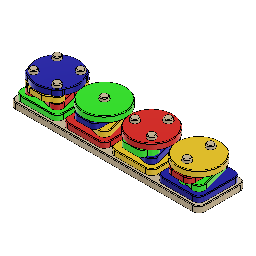
SHAPESpuzzle (Autodesk Fusion 360 design; units mm, degrees)
Autodesk Fusion 360 part; units mm, degrees
note: some values were not read from the file. Chosen so that the rebuilt part matches the saved one: which pieces of a blend or face edit are solid. Set by a fixed rule: which sketch regions a step uses.
sketch "baseboard" plane through (0, 0, 0) normal (0, 0, 1) x (1, 0, 0) in component "base"
  line L0 (160, 40) -> (-160, 40)
  line L1 (-160, 40) -> (-160, -40)
  line L2 (-160, -40) -> (160, -40)
  line L3 (160, -40) -> (160, 40)
  line L4 (160, 40) -> (-160, -40) construction
  line L5 (-160, 40) -> (160, -40) construction
  line L6 (80, 40) -> (-80, 40) construction
  line L7 (-80, 40) -> (-80, -40) construction
  line L8 (-80, -40) -> (80, -40) construction
  line L9 (80, -40) -> (80, 40) construction
  line L10 (80, 40) -> (-80, -40) construction
  line L11 (-80, 40) -> (80, -40) construction
  line L12 (0, 40) -> (0, -40) construction
  line L13 (80, 40) -> (160, -40) construction
  line L14 (160, 40) -> (80, -40) construction
  line L15 (80, -40) -> (0, 40) construction
  line L16 (0, 40) -> (-80, -40) construction
  line L17 (-80, -40) -> (-160, 40) construction
  line L18 (-160, -40) -> (-80, 40) construction
  line L19 (-80, 40) -> (0, -40) construction
  line L20 (0, -40) -> (80, 40) construction
  circle A0 centre (-40, 0) radius 6
  line L21 (120, 40) -> (120, -40)
  circle A1 centre (120, 20) radius 6
  circle A2 centre (120, -20) radius 6
  circle A3 centre (-100, -20) radius 6
  circle A4 centre (-100, 20) radius 6
  circle A5 centre (-140, 20) radius 6
  circle A6 centre (-140, -20) radius 6
  circle A7 centre (56.3299, -16.3299) radius 6
  circle A8 centre (45.9772, 22.3071) radius 6
  circle A9 centre (17.6929, -5.9772) radius 6
  point P0 (120, 0)
  point P1 (-120, 0)
  point P2 (40, 0)
  dimension "d1" = 320
  dimension "d2" = 80
  dimension "d3" = 160
  dimension "d4" = 80
  dimension "d7" = 12
  dimension "d8" = 40
  dimension "d9" = 12
  dimension "d11" = 20
  dimension "d13" = 360
  dimension "d26" = 12
  dimension "d27" = 28.2843
  dimension "d29" = 360
  dimension "d89" = 12
  dimension "d90" = 23.094
  dimension "d92" = 360
  constraint horizontal L0
  constraint perpendicular L0 L1
  constraint parallel L0 L2
  constraint parallel L1 L3
  constraint coincident L4 origin
  constraint coincident L5 origin
  constraint horizontal L6
  constraint perpendicular L6 L7
  constraint parallel L6 L8
  constraint parallel L7 L9
  constraint coincident L10 origin
  constraint coincident L11 origin
  constraint midpoint L0 L12.start
  constraint midpoint L2 L12.end
  constraint midpoint L19 A0.centre
  constraint coincident L0 L21.start
  constraint coincident L2 L21.end
  constraint perpendicular L2 L21
  constraint coincident L21 A1.centre
  constraint midpoint L13 P0
  constraint midpoint L17 P1
  constraint midpoint L15 P2
  constraint coincident L17 A3.centre
  constraint coincident L15 A7.centre
  measures "d1" distance of L1.end L2.end
  measures "d2" distance of L0.end L1.end
  measures "d3" distance of L7.end L8.end
  measures "d4" distance of L6.end L7.end
  measures "d7" diameter of A0
  measures "d8" distance of L6.start L21.start
  measures "d9" diameter of A1
  measures "d11" distance of A1.centre P0
  measures "d26" diameter of A3
  measures "d27" distance of P1 A3.centre
  measures "d89" diameter of A7
  measures "d90" distance of P2 A7.centre
extrude "Extrude1" add sketch "baseboard" along normal blind 10 contours L0 L2 L3 L21 A1 A2 | L0 L1 L2 L21 A1 A2 makes body 1 in component "base"
fillet "Fillet1" radius 10 4 edges at (-160, 40, 5) (-160, -40, 5) (160, -40, 5) (160, 40, 5) on bodies 1 in component "base"
ref_plane "WorkPlane2" through (0, 0, -40) normal (0, 0, 1) x (1, 0, 0) in component "base"
sketch "laser cutting" plane through (0, 0, -40) normal (0, 0, 1) x (1, 0, 0) in component "base"
  arc A0 (160, 30) -> (150, 40) centre (150, 30) ccw
  line L0 (150, 40) -> (-150, 40)
  arc A1 (-150, 40) -> (-160, 30) centre (-150, 30) ccw
  line L1 (-160, 30) -> (-160, -30)
  arc A2 (-160, -30) -> (-150, -40) centre (-150, -30) ccw
  line L2 (-150, -40) -> (150, -40)
  arc A3 (150, -40) -> (160, -30) centre (150, -30) ccw
  line L3 (160, -30) -> (160, 30)
  circle A4 centre (-100, 20) radius 6
  circle A5 centre (-40, 0) radius 6
  circle A6 centre (-140, 20) radius 6
  circle A7 centre (120, -20) radius 6
  circle A8 centre (120, 20) radius 6
  circle A9 centre (-100, -20) radius 6
  circle A10 centre (-140, -20) radius 6
  circle A11 centre (17.6929, -5.9772) radius 6
  circle A12 centre (45.9772, 22.3071) radius 6
  circle A13 centre (56.3299, -16.3299) radius 6
chamfer "Chamfer2" distance 1 angle 45 8 edges at (160, 0, 10) (157.0711, 37.0711, 10) (0, 40, 10) (-157.0711, 37.0711, 10) (-160, 0, 10) (-157.0711, -37.0711, 10) (0, -40, 10) (157.0711, -37.0711, 10) on bodies 1 in component "base"
extrude "Extrude1'" add sketch "baseboard" along normal blind 55 separate body contours L21 A1 | L21 A1 | L21 A2 | L21 A2 | A0 | A3 | A4 | A5 | A6 | A7 | A8 | A9 makes body 2 at (-94.0298, 19.4026, 18.3333) makes body 3 at (-34.0298, -0.5974, 18.3333) makes body 4 at (-94.0298, -20.5974, 18.3333) makes body 5 at (125.9925, -20.2991, 18.3333) makes body 6 at (-138.375, 25.7757, 36.6667) makes body 7 at (-142.7373, -25.3392, 18.3333) makes body 8 at (125.9925, 19.7009, 18.3333) makes body 9 at (23.6631, -6.5746, 18.3333) makes body 10 at (62.3001, -16.9273, 18.3333) makes body 11 at (51.9474, 21.7097, 18.3333) in component "pins"
chamfer "Chamfer1" distance 1 angle 45 10 edges at (50.736, -18.4996, 55) (12.0989, -8.1469, 55) (40.3832, 20.1374, 55) (114.406, -22.1697, 55) (-145.594, -22.1697, 55) (-145.594, 17.8303, 55) (-45.594, -2.1697, 55) (-105.594, 17.8303, 55) (-105.594, -22.1697, 55) (114.406, 17.8303, 55) on bodies 2 3 4 5 6 7 8 9 10 11 in component "pins"
sketch "squareSketch" plane through (0, 0, 0) normal (0, 0, 1) x (1, 0, 0) in component "square4"
  line L0 (-160, 40) -> (-80, 40)
  line L1 (-80, 40) -> (-80, -40)
  line L2 (-80, -40) -> (-160, -40)
  line L3 (-160, -40) -> (-160, 40)
  constraint horizontal L0
  constraint vertical L1
  constraint horizontal L2
  constraint vertical L3
extrude "Extrude1''" add sketch "squareSketch" along normal blind 10 separate body makes body 12 in component "square4"
extrude "Extrude2" cut sketch "squareSketch" along normal blind 10 thin wall 4 inside bodies 12 in component "square4"
extrude "Extrude3" cut sketch "baseboard" along normal blind 10 contours A3 | A4 | A5 | A6 bodies 12 in component "square4"
fillet "Fillet1'" radius 10 4 edges at (-84, -36, 5) (-84, 36, 5) (-156, -36, 5) (-156, 36, 5) on bodies 12 in component "square4"
chamfer "Chamfer1'" distance 1 angle 45 16 edges at (-153.0711, 33.0711, 10) (-120, 36, 10) (-86.9289, 33.0711, 10) (-84, 0, 10) (-86.9289, -33.0711, 10) (-120, -36, 10) (-153.0711, -33.0711, 10) (-156, 0, 10) (-153.0711, 33.0711, 0) (-156, 0, 0) (-153.0711, -33.0711, 0) (-120, -36, 0) (-86.9289, -33.0711, 0) (-84, 0, 0) (-86.9289, 33.0711, 0) (-120, 36, 0) on bodies 12 in component "square4"
chamfer "Chamfer1'" distance 1 angle 45 8 edges at (-145.594, 22.1697, 10) (-145.594, -17.8303, 10) (-145.594, -22.1697, 0) (-105.594, 22.1697, 10) (-105.594, 17.8303, 0) (-145.594, 17.8303, 0) (-105.594, -17.8303, 10) (-105.594, -22.1697, 0) on bodies 12 in component "square4"
sketch "Sketch1" plane through (0, 0, 0) normal (0, 0, 1) x (1, 0, 0) in component "circle1"
  circle A0 centre (-40, 0) radius 36
  dimension "d236" = 1
  dimension "d237" = 1
  measures "d54" diameter of A0
extrude "Extrude1'''" add sketch "Sketch1" along normal blind 10 separate body makes body 13 in component "circle1"
extrude "Extrude2'" cut sketch "baseboard" along normal blind 10 contours A0 bodies 13 in component "circle1"
chamfer "Chamfer1''" distance 1 angle 45 4 edges at (-73.5638, -13.0182, 0) (-73.5638, -13.0182, 10) (-45.594, 2.1697, 10) (-45.594, -2.1697, 0) on bodies 13 in component "circle1"
sketch "triangleSketch" plane through (0, 0, 0) normal (0, 0, 1) x (1, 0, 0) in component "triangle3"
  circle A0 centre (40, 0) radius 48
  line L0 (40, 0) -> (-6.3644, -12.4233) construction
  line L1 (40, 0) -> (73.9411, -33.9411) construction
  line L2 (40, 0) -> (52.4233, 46.3644) construction
  line L3 (-6.3644, -12.4233) -> (73.9411, -33.9411)
  line L4 (52.4233, 46.3644) -> (73.9411, -33.9411)
  line L5 (52.4233, 46.3644) -> (-6.3644, -12.4233)
  point P0 (52.4233, 46.3644)
  point P1 (40, 0)
  dimension "d66" = 96
  constraint coincident P1 A0.centre
  constraint coincident A0 L0.end
  constraint coincident A0 L1.end
  constraint coincident A0 P0
  constraint coincident P0 L2.end
  measures "d66" diameter of A0
extrude "Extrude2''" add sketch "triangleSketch" along normal blind 10 separate body contours L3 L4 L5 makes body 14 in component "triangle3"
extrude "Extrude3'" cut sketch "baseboard" along normal blind 10 contours A7 | A8 | A9 bodies 14 in component "triangle3"
fillet "Fillet1''" radius 10 3 edges at (-6.3644, -12.4233, 5) (73.9411, -33.9411, 5) (52.4233, 46.3644, 5) on bodies 14 in component "triangle3"
chamfer "Chamfer1'''" distance 1 angle 45 18 edges at (33.7883, -23.1822, 10) (66.8701, -26.8701, 10) (63.1822, 6.2117, 10) (49.8351, 36.7052, 10) (23.0294, 16.9706, 10) (3.2948, -9.8351, 10) (66.8701, -26.8701, 0) (63.1822, 6.2117, 0) (49.8351, 36.7052, 0) (23.0294, 16.9706, 0) (3.2948, -9.8351, 0) (33.7883, -23.1822, 0) (40.3832, 24.4768, 10) (50.736, -14.1602, 10) (12.0989, -3.8075, 10) (50.736, -18.4996, 0) (12.0989, -8.1469, 0) (40.3832, 20.1374, 0) on bodies 14 in component "triangle3"
sketch "Sketch2" plane through (0, 0, 0) normal (0, 0, 1) x (1, 0, 0) in component "rectangle2"
  line L0 (140, 36) -> (100, 36)
  line L1 (100, 36) -> (100, -36)
  line L2 (100, -36) -> (140, -36)
  line L3 (140, -36) -> (140, 36)
  line L4 (140, 36) -> (100, -36) construction
  line L5 (100, 36) -> (140, -36) construction
  point P0 (120, 0)
  dimension "d79" = 40
  dimension "d80" = 72
  constraint horizontal L0
  constraint perpendicular L0 L1
  constraint parallel L0 L2
  constraint parallel L1 L3
  constraint coincident L4 P0
  constraint coincident L5 P0
  measures "d79" distance of L1.end L2.end
  measures "d80" distance of L0.end L1.end
extrude "Extrude2'''" add sketch "Sketch2" along normal blind 10 separate body makes body 15 in component "rectangle2"
extrude "Extrude3''" cut sketch "baseboard" along normal blind 10 contours L21 A1 | L21 A1 | L21 A2 | L21 A2 bodies 15 in component "rectangle2"
fillet "Fillet1'''" radius 10 4 edges at (100, -36, 5) (140, -36, 5) (140, 36, 5) (100, 36, 5) on bodies 15 in component "rectangle2"
chamfer "Chamfer1''''" distance 1 angle 45 4 edges at (114.406, 22.1697, 10) (114.406, -17.8303, 10) (114.406, 17.8303, 0) (114.406, -22.1697, 0) on bodies 15 in component "rectangle2"
chamfer "Chamfer1''''" distance 1 angle 45 16 edges at (140, 0, 10) (137.0711, 33.0711, 10) (120, 36, 10) (102.9289, 33.0711, 10) (100, 0, 10) (102.9289, -33.0711, 10) (120, -36, 10) (137.0711, -33.0711, 10) (120, -36, 0) (137.0711, -33.0711, 0) (140, 0, 0) (137.0711, 33.0711, 0) (120, 36, 0) (102.9289, 33.0711, 0) (100, 0, 0) (102.9289, -33.0711, 0) on bodies 15 in component "rectangle2"
sketch "Sketch1 (2)" plane through (0, 0, 0) normal (0, 0, 1) x (1, 0, 0) in component "circle2"
  circle A0 centre (120, 0) radius 36
  dimension "d93" = 72
  measures "d93" diameter of A0
extrude "Extrude1''''" add sketch "Sketch1 (2)" along normal blind 10 separate body makes body 16 in component "circle2"
extrude "Extrude2''''" cut sketch "baseboard" along normal blind 10 contours L21 A1 | L21 A1 | L21 A2 | L21 A2 bodies 16 in component "circle2"
chamfer "Chamfer1'''''" distance 1 angle 45 2 edges at (86.4362, -13.0182, 0) (86.4362, -13.0182, 10) on bodies 16 in component "circle2"
chamfer "Chamfer1'''''" distance 1 angle 45 4 edges at (114.406, 22.1697, 10) (114.406, -17.8303, 10) (114.406, -22.1697, 0) (114.406, 17.8303, 0) on bodies 16 in component "circle2"
sketch "Sketch2 (2)" plane through (0, 0, 0) normal (0, 0, 1) x (1, 0, 0) in component "square2"
  line L0 (160, 40) -> (80, 40)
  line L1 (80, 40) -> (80, -40)
  line L2 (80, -40) -> (160, -40)
  line L3 (160, -40) -> (160, 40)
  line L4 (160, 40) -> (80, -40) construction
  line L5 (80, 40) -> (160, -40) construction
  point P0 (120, 0)
  dimension "d102" = 80
  dimension "d103" = 80
  constraint horizontal L0
  constraint perpendicular L0 L1
  constraint parallel L0 L2
  constraint parallel L1 L3
  constraint coincident L4 P0
  constraint coincident L5 P0
  measures "d102" distance of L1.end L2.end
  measures "d103" distance of L0.end L1.end
extrude "Extrude1'''''" add sketch "Sketch2 (2)" along normal blind 10 separate body makes body 17 in component "square2"
extrude "Extrude2'''''" cut sketch "Sketch2 (2)" along normal blind 10 thin wall 4 inside bodies 17 in component "square2"
extrude "Extrude3'''" cut sketch "baseboard" along normal blind 10 contours L21 A1 | L21 A1 | L21 A2 | L21 A2 bodies 17 in component "square2"
fillet "Fillet1''''" radius 10 4 edges at (156, -36, 5) (156, 36, 5) (84, -36, 5) (84, 36, 5) on bodies 17 in component "square2"
chamfer "Chamfer1''''''" distance 1 angle 45 4 edges at (114.406, 22.1697, 10) (114.406, -17.8303, 10) (114.406, -22.1697, 0) (114.406, 17.8303, 0) on bodies 17 in component "square2"
chamfer "Chamfer1''''''" distance 1 angle 45 16 edges at (120, -36, 10) (153.0711, -33.0711, 10) (156, 0, 10) (153.0711, 33.0711, 10) (120, 36, 10) (86.9289, 33.0711, 10) (84, 0, 10) (86.9289, -33.0711, 10) (120, -36, 0) (86.9289, -33.0711, 0) (84, 0, 0) (86.9289, 33.0711, 0) (120, 36, 0) (153.0711, 33.0711, 0) (156, 0, 0) (153.0711, -33.0711, 0) on bodies 17 in component "square2"
sketch "Sketch1 (3)" plane through (0, 0, 0) normal (0, 0, 1) x (1, 0, 0) in component "circle4"
  circle A0 centre (-120, 0) radius 36
  dimension "d115" = 72
  measures "d115" diameter of A0
extrude "Extrude1''''''" add sketch "Sketch1 (3)" along normal blind 10 separate body makes body 18 in component "circle4"
extrude "Extrude2''''''" cut sketch "baseboard" along normal blind 10 contours A3 | A4 | A5 | A6 bodies 18 in component "circle4"
extrude "Extrude3''''" add sketch "baseboard" along normal blind 10 thin wall 4 outside contours A3 | A4 | A5 | A6 bodies 18 in component "circle4"
fillet "Fillet1'''''" radius 5 8 edges at (-100.0995, -29.9995, 5) (-90.0005, -19.9005, 5) (-90.0005, 19.9005, 5) (-139.9005, -29.9995, 5) (-149.9995, -19.9005, 5) (-149.9995, 19.9005, 5) (-139.9005, 29.9995, 5) (-100.0995, 29.9995, 5) on bodies 18 in component "circle4"
chamfer "Chamfer1'''''''" distance 1 angle 45 8 edges at (-105.594, -17.8303, 10) (-145.594, -17.8303, 10) (-145.594, 22.1697, 10) (-105.594, 22.1697, 10) (-105.594, -22.1697, 0) (-145.594, -22.1697, 0) (-145.594, 17.8303, 0) (-105.594, 17.8303, 0) on bodies 18 in component "circle4"
chamfer "Chamfer1'''''''" distance 1 angle 45 2 edges at (-153.5638, -13.0182, 0) (-153.5638, -13.0182, 10) on bodies 18 in component "circle4"
sketch "Sketch2 (3)" plane through (0, 0, 0) normal (0, 0, 1) x (1, 0, 0) in component "rectangle1"
  line L0 (-20, 36) -> (-60, 36)
  line L1 (-60, 36) -> (-60, -36)
  line L2 (-60, -36) -> (-20, -36)
  line L3 (-20, -36) -> (-20, 36)
  line L4 (-20, 36) -> (-60, -36) construction
  line L5 (-60, 36) -> (-20, -36) construction
  point P0 (-40, 0)
  dimension "d126" = 40
  dimension "d127" = 72
  constraint horizontal L0
  constraint perpendicular L0 L1
  constraint parallel L0 L2
  constraint parallel L1 L3
  constraint coincident L4 P0
  constraint coincident L5 P0
  measures "d126" distance of L1.end L2.end
  measures "d127" distance of L0.end L1.end
extrude "Extrude1'''''''" add sketch "Sketch2 (3)" along normal blind 10 separate body makes body 19 in component "rectangle1"
extrude "Extrude2'''''''" cut sketch "baseboard" along normal blind 10 contours A0 bodies 19 in component "rectangle1"
fillet "Fillet1''''''" radius 10 4 edges at (-60, 36, 5) (-20, 36, 5) (-20, -36, 5) (-60, -36, 5) on bodies 19 in component "rectangle1"
chamfer "Chamfer1''''''''" distance 1 angle 45 16 edges at (-20, 0, 10) (-22.9289, 33.0711, 10) (-40, 36, 10) (-57.0711, 33.0711, 10) (-60, 0, 10) (-57.0711, -33.0711, 10) (-40, -36, 10) (-22.9289, -33.0711, 10) (-20, 0, 0) (-22.9289, 33.0711, 0) (-40, 36, 0) (-57.0711, 33.0711, 0) (-60, 0, 0) (-57.0711, -33.0711, 0) (-40, -36, 0) (-22.9289, -33.0711, 0) on bodies 19 in component "rectangle1"
chamfer "Chamfer1''''''''" distance 1 angle 45 2 edges at (-45.594, 2.1697, 10) (-45.594, -2.1697, 0) on bodies 19 in component "rectangle1"
sketch "Sketch1 (4)" plane through (0, 0, 0) normal (0, 0, 1) x (1, 0, 0) in component "rectangle3"
  line L0 (60, -36) -> (20, -36)
  line L1 (20, -36) -> (20, 36)
  line L2 (20, 36) -> (60, 36)
  line L3 (60, 36) -> (60, -36)
  line L4 (60, -36) -> (20, 36) construction
  line L5 (20, -36) -> (60, 36) construction
  point P0 (40, 0)
  dimension "d136" = 40
  dimension "d137" = 72
  constraint horizontal L0
  constraint perpendicular L0 L1
  constraint parallel L0 L2
  constraint parallel L1 L3
  constraint coincident L4 P0
  constraint coincident L5 P0
  measures "d136" distance of L1.end L2.end
  measures "d137" distance of L0.end L1.end
extrude "Extrude1''''''''" add sketch "Sketch1 (4)" along normal blind 10 separate body makes body 20 in component "rectangle3"
extrude "Extrude3'''''" add sketch "baseboard" along normal blind 10 thin wall 4 outside contours A7 | A9 bodies 20 in component "rectangle3"
fillet "Fillet1'''''''" radius 10 4 edges at (20, 36, 5) (60, 36, 5) (20, -36, 5) (60, -36, 5) on bodies 20 in component "rectangle3"
fillet "Fillet1'''''''" radius 5 4 edges at (60, -25.6321, 5) (60, -7.0277, 5) (20, 3.7531, 5) (20, -15.7074, 5) on bodies 20 in component "rectangle3"
sketch "Sketch1 (5)" plane through (0, 0, 0) normal (0, 0, 1) x (1, 0, 0) in component "square1"
  line L0 (-4, 36) -> (-76, 36)
  line L1 (-76, 36) -> (-76, -36)
  line L2 (-76, -36) -> (-4, -36)
  line L3 (-4, -36) -> (-4, 36)
  line L4 (-4, 36) -> (-76, -36) construction
  line L5 (-76, 36) -> (-4, -36) construction
  point P0 (-40, 0)
  dimension "d153" = 72
  dimension "d154" = 72
  constraint horizontal L0
  constraint perpendicular L0 L1
  constraint parallel L0 L2
  constraint parallel L1 L3
  constraint coincident L4 P0
  constraint coincident L5 P0
  measures "d153" distance of L1.end L2.end
  measures "d154" distance of L0.end L1.end
extrude "Extrude1'''''''''" add sketch "Sketch1 (5)" along normal blind 10 separate body makes body 21 in component "square1"
extrude "Extrude2''''''''" cut sketch "baseboard" along normal blind 10 contours A0 bodies 21 in component "square1"
fillet "Fillet1''''''''" radius 10 4 edges at (-4, -36, 5) (-4, 36, 5) (-76, -36, 5) (-76, 36, 5) on bodies 21 in component "square1"
chamfer "Chamfer1'''''''''" distance 1 angle 45 16 edges at (-40, 36, 10) (-73.0711, 33.0711, 10) (-76, 0, 10) (-73.0711, -33.0711, 10) (-40, -36, 10) (-6.9289, -33.0711, 10) (-4, 0, 10) (-6.9289, 33.0711, 10) (-40, 36, 0) (-73.0711, 33.0711, 0) (-76, 0, 0) (-73.0711, -33.0711, 0) (-40, -36, 0) (-6.9289, -33.0711, 0) (-4, 0, 0) (-6.9289, 33.0711, 0) on bodies 21 in component "square1"
chamfer "Chamfer1'''''''''" distance 1 angle 45 2 edges at (-45.594, 2.1697, 10) (-45.594, -2.1697, 0) on bodies 21 in component "square1"
sketch "Sketch1 (6)" plane through (0, 0, 0) normal (0, 0, 1) x (1, 0, 0) in component "triangle4"
  circle A0 centre (-120, 0) radius 48
  line L0 (-120, 0) -> (-86.0589, -33.9411) construction
  line L1 (-80, -40) -> (-160, 40)
  line L2 (-120, 0) -> (-107.5767, 46.3644) construction
  line L3 (-120, 0) -> (-166.3644, -12.4233) construction
  line L4 (-107.5767, 46.3644) -> (-86.0589, -33.9411)
  line L5 (-166.3644, -12.4233) -> (-86.0589, -33.9411)
  line L6 (-166.3644, -12.4233) -> (-107.5767, 46.3644)
  point P0 (-120, 0)
  dimension "d163" = 96
  dimension "d165" = 360
  constraint coincident P0 A0.centre
  constraint coincident A0 L0.end
  constraint parallel L0 L1
  measures "d163" diameter of A0
extrude "Extrude1''''''''''" add sketch "Sketch1 (6)" along normal blind 10 separate body contours L1 L4 L6 | L1 L5 L6 makes body 22 in component "triangle4"
extrude "Extrude2'''''''''" cut sketch "baseboard" along normal blind 10 contours A3 | A4 | A5 | A6 bodies 22 in component "triangle4"
extrude "Extrude3''''''" add sketch "baseboard" along normal blind 10 thin wall 4 outside contours A4 | A5 | A6 bodies 22 in component "triangle4"
fillet "Fillet1'''''''''" radius 10 3 edges at (-86.0589, -33.9411, 5) (-166.3644, -12.4233, 5) (-107.5767, 46.3644, 5) on bodies 22 in component "triangle4"
fillet "Fillet1'''''''''" radius 5 6 edges at (-130.2245, -22.107, 5) (-97.893, 10.2245, 5) (-149.5193, -16.9369, 5) (-143.3598, 10.5813, 5) (-103.0631, 29.5193, 5) (-130.5813, 23.3598, 5) on bodies 22 in component "triangle4"
chamfer "Chamfer1''''''''''" distance 1 angle 45 32 edges at (-93.6584, -5.5794, 10) (-96.605, 9.1591, 10) (-90.3407, 22.5882, 10) (-101.9415, 30.7091, 10) (-111.033, 37.3831, 10) (-122.8892, 31.0519, 10) (-129.7923, 26.102, 10) (-147.0711, 27.0711, 10) (-146.102, 9.7923, 10) (-150.841, 3.1001, 10) (-156.9819, -8.3769, 10) (-150.6235, -17.5464, 10) (-142.8078, -29.5977, 10) (-129.1591, -23.395, 10) (-114.4206, -26.3416, 10) (-93.1299, -26.8701, 10) (-93.6584, -5.5794, 0) (-93.1299, -26.8701, 0) (-114.4206, -26.3416, 0) (-129.1591, -23.395, 0) (-142.8078, -29.5977, 0) (-150.6235, -17.5464, 0) (-156.9819, -8.3769, 0) (-150.841, 3.1001, 0) (-146.102, 9.7923, 0) (-147.0711, 27.0711, 0) (-129.7923, 26.102, 0) (-122.8892, 31.0519, 0) (-111.033, 37.3831, 0) (-101.9415, 30.7091, 0) (-90.3407, 22.5882, 0) (-96.605, 9.1591, 0) on bodies 22 in component "triangle4"
chamfer "Chamfer1''''''''''" distance 1 angle 45 8 edges at (-105.594, -17.8303, 10) (-145.594, -17.8303, 10) (-145.594, 22.1697, 10) (-105.594, 22.1697, 10) (-105.594, 17.8303, 0) (-145.594, 17.8303, 0) (-105.594, -22.1697, 0) (-145.594, -22.1697, 0) on bodies 22 in component "triangle4"
sketch "Sketch1 (7)" plane through (0, 0, 0) normal (0, 0, 1) x (1, 0, 0) in component "circle3"
  circle A0 centre (40, 0) radius 36
  dimension "d179" = 72
  measures "d179" diameter of A0
extrude "Extrude1'''''''''''" add sketch "Sketch1 (7)" along normal blind 10 separate body makes body 23 in component "circle3"
extrude "Extrude2''''''''''" cut sketch "baseboard" along normal blind 10 contours A7 | A8 | A9 bodies 23 in component "circle3"
chamfer "Chamfer1'''''''''''" distance 1 angle 45 2 edges at (6.4362, -13.0182, 10) (6.4362, -13.0182, 0) on bodies 23 in component "circle3"
chamfer "Chamfer1'''''''''''" distance 1 angle 45 6 edges at (40.3832, 24.4768, 10) (50.736, -14.1602, 10) (12.0989, -3.8075, 10) (50.736, -18.4996, 0) (12.0989, -8.1469, 0) (40.3832, 20.1374, 0) on bodies 23 in component "circle3"
sketch "Sketch1 (8)" plane through (0, 0, 0) normal (0, 0, 1) x (1, 0, 0) in component "triangle2"
  circle A0 centre (119.9685, 0.0315) radius 48
  line L0 (119.9685, 0.0315) -> (153.9096, -33.9096) construction
  line L1 (80, 40) -> (160, -40)
  line L2 (119.9685, 0.0315) -> (132.3918, 46.396) construction
  line L3 (119.9685, 0.0315) -> (73.604, -12.3918) construction
  line L4 (153.9096, -33.9096) -> (73.604, -12.3918)
  line L5 (73.604, -12.3918) -> (132.3918, 46.396)
  line L6 (132.3918, 46.396) -> (153.9096, -33.9096)
  point P0 (120, 0)
  dimension "d186" = 96
  dimension "d188" = 360
  constraint coincident A0.centre L0.start
  constraint coincident A0 L0.end
  constraint parallel L0 L1
  constraint coincident L0 P0
  measures "d186" diameter of A0
extrude "Extrude1''''''''''''" add sketch "Sketch1 (8)" along normal blind 10 separate body contours L1 L5 L6 | L1 L4 L5 makes body 24 in component "triangle2"
extrude "Extrude2'''''''''''" cut sketch "baseboard" along normal blind 10 contours L21 A1 | L21 A1 | L21 A2 | L21 A2 bodies 24 in component "triangle2"
extrude "Extrude3'''''''" add sketch "baseboard" along normal blind 10 thin wall 4 outside contours L21 A2 | L21 A2 bodies 24 in component "triangle2"
fillet "Fillet1''''''''''" radius 10 3 edges at (153.9096, -33.9096, 5) (73.604, -12.3918, 5) (132.3918, 46.396, 5) on bodies 24 in component "triangle2"
fillet "Fillet1''''''''''" radius 5 2 edges at (110.2473, -22.2103, 5) (127.3409, -26.7905, 5) on bodies 24 in component "triangle2"
chamfer "Chamfer1''''''''''''" distance 1 angle 45 20 edges at (133.5292, -28.4487, 10) (146.8385, -26.8385, 10) (143.1507, 6.2432, 10) (129.8036, 36.7367, 10) (102.9979, 17.0021, 10) (83.2633, -9.8036, 10) (99.0217, -19.2024, 10) (109.626, -22.5272, 10) (117.4118, -29.6593, 10) (127.7205, -27.3756, 10) (146.8385, -26.8385, 0) (143.1507, 6.2432, 0) (129.8036, 36.7367, 0) (102.9979, 17.0021, 0) (83.2633, -9.8036, 0) (99.0217, -19.2024, 0) (109.626, -22.5272, 0) (117.4118, -29.6593, 0) (127.7205, -27.3756, 0) (133.5292, -28.4487, 0) on bodies 24 in component "triangle2"
chamfer "Chamfer1''''''''''''" distance 1 angle 45 4 edges at (114.406, 22.1697, 10) (114.406, -17.8303, 10) (114.406, -22.1697, 0) (114.406, 17.8303, 0) on bodies 24 in component "triangle2"
sketch "Sketch1 (9)" plane through (0, 0, 0) normal (0, 0, 1) x (1, 0, 0) in component "square3"
  line L0 (76, 36) -> (4, 36)
  line L1 (4, 36) -> (4, -36)
  line L2 (4, -36) -> (76, -36)
  line L3 (76, -36) -> (76, 36)
  line L4 (76, 36) -> (4, -36) construction
  line L5 (4, 36) -> (76, -36) construction
  point P0 (40, 0)
  dimension "d202" = 72
  dimension "d203" = 72
  constraint horizontal L0
  constraint perpendicular L0 L1
  constraint parallel L0 L2
  constraint parallel L1 L3
  constraint coincident L4 P0
  constraint coincident L5 P0
  measures "d202" distance of L1.end L2.end
  measures "d203" distance of L0.end L1.end
extrude "Extrude1'''''''''''''" add sketch "Sketch1 (9)" along normal blind 10 separate body makes body 25 in component "square3"
extrude "Extrude2''''''''''''" cut sketch "baseboard" along normal blind 10 contours A7 | A8 | A9 bodies 25 in component "square3"
fillet "Fillet1'''''''''''" radius 10 4 edges at (76, -36, 5) (4, -36, 5) (76, 36, 5) (4, 36, 5) on bodies 25 in component "square3"
chamfer "Chamfer1'''''''''''''" distance 1 angle 45 16 edges at (40, -36, 0) (73.0711, -33.0711, 0) (76, 0, 0) (73.0711, 33.0711, 0) (40, 36, 0) (6.9289, 33.0711, 0) (4, 0, 0) (6.9289, -33.0711, 0) (40, -36, 10) (73.0711, -33.0711, 10) (76, 0, 10) (73.0711, 33.0711, 10) (40, 36, 10) (6.9289, 33.0711, 10) (4, 0, 10) (6.9289, -33.0711, 10) on bodies 25 in component "square3"
chamfer "Chamfer1'''''''''''''" distance 1 angle 45 6 edges at (50.736, -18.4996, 0) (40.3832, 20.1374, 0) (12.0989, -8.1469, 0) (50.736, -14.1602, 10) (40.3832, 24.4768, 10) (12.0989, -3.8075, 10) on bodies 25 in component "square3"
sketch "Sketch1 (10)" plane through (0, 0, 0) normal (0, 0, 1) x (1, 0, 0) in component "triangle1"
  circle A0 centre (-40, 0) radius 48 construction
  line L0 (-40, 0) -> (-6.0589, -33.9411) construction
  line L1 (-80, 40) -> (0, -40)
  line L2 (-40, 0) -> (-27.5767, 46.3644) construction
  line L3 (-40, 0) -> (-86.3644, -12.4233) construction
  line L4 (-86.3644, -12.4233) -> (-27.5767, 46.3644)
  line L5 (-6.0589, -33.9411) -> (-86.3644, -12.4233)
  line L6 (-27.5767, 46.3644) -> (-6.0589, -33.9411)
  point P0 (-40, 0)
  dimension "d212" = 96
  dimension "d214" = 360
  constraint coincident P0 A0.centre
  constraint coincident A0 L0.end
  constraint parallel L0 L1
  measures "d212" diameter of A0
extrude "Extrude1''''''''''''''" add sketch "Sketch1 (10)" along normal blind 10 separate body makes body 26 in component "triangle1"
extrude "Extrude2'''''''''''''" cut sketch "baseboard" along normal blind 10 contours A0 bodies 26 in component "triangle1"
fillet "Fillet1''''''''''''" radius 10 3 edges at (-86.3644, -12.4233, 5) (-6.0589, -33.9411, 5) (-27.5767, 46.3644, 5) on bodies 26 in component "triangle1"
chamfer "Chamfer1''''''''''''''" distance 1 angle 45 12 edges at (-13.1299, -26.8701, 10) (-46.2117, -23.1822, 10) (-76.7052, -9.8351, 10) (-56.9706, 16.9706, 10) (-30.1649, 36.7052, 10) (-16.8178, 6.2117, 10) (-13.1299, -26.8701, 0) (-16.8178, 6.2117, 0) (-30.1649, 36.7052, 0) (-56.9706, 16.9706, 0) (-76.7052, -9.8351, 0) (-46.2117, -23.1822, 0) on bodies 26 in component "triangle1"
chamfer "Chamfer1''''''''''''''" distance 1 angle 45 2 edges at (-45.594, 2.1697, 10) (-45.594, -2.1697, 0) on bodies 26 in component "triangle1"
sketch "Sketch1 (11)" plane through (0, 0, 0) normal (0, 0, 1) x (1, 0, 0) in component "rectangle4"
  line L0 (-100, 36) -> (-140, 36)
  line L1 (-140, 36) -> (-140, -36)
  line L2 (-140, -36) -> (-100, -36)
  line L3 (-100, -36) -> (-100, 36)
  line L4 (-100, 36) -> (-140, -36) construction
  line L5 (-140, 36) -> (-100, -36) construction
  point P0 (-120, 0)
  dimension "d223" = 40
  dimension "d224" = 72
  constraint horizontal L0
  constraint perpendicular L0 L1
  constraint parallel L0 L2
  constraint parallel L1 L3
  constraint coincident L4 P0
  constraint coincident L5 P0
  measures "d223" distance of L1.end L2.end
  measures "d224" distance of L0.end L1.end
extrude "Extrude1'''''''''''''''" add sketch "Sketch1 (11)" along normal blind 10 separate body makes body 27 in component "rectangle4"
extrude "Extrude2''''''''''''''" cut sketch "baseboard" along normal blind 10 contours A3 | A4 | A5 | A6 bodies 27 in component "rectangle4"
fillet "Fillet1'''''''''''''" radius 10 4 edges at (-100, -36, 5) (-140, -36, 5) (-100, 36, 5) (-140, 36, 5) on bodies 27 in component "rectangle4"
extrude "Extrude3''''''''" add sketch "baseboard" along normal blind 10 thin wall 4 outside contours A3 | A4 | A5 | A6 bodies 27 in component "rectangle4"
fillet "Fillet2" radius 5 8 edges at (-100.8202, -29.9663, 5) (-100, 10, 5) (-100, -10, 5) (-100.8202, 29.9663, 5) (-139.1798, 29.9663, 5) (-140, -10, 5) (-140, 10, 5) (-139.1798, -29.9663, 5) on bodies 27 in component "rectangle4"
chamfer "Chamfer1'''''''''''''''" distance 1 angle 45 40 edges at (-100, 0, 10) (-99.0825, 8.7446, 10) (-90.0493, 20.9917, 10) (-100.462, 30.5633, 10) (-105.4726, 34.9164, 10) (-120, 36, 10) (-134.5274, 34.9164, 10) (-139.538, 30.5633, 10) (-149.9507, 20.9917, 10) (-140.9175, 8.7446, 10) (-140, 0, 10) (-140.9175, -8.7446, 10) (-149.9507, -20.9917, 10) (-139.538, -30.5633, 10) (-134.5274, -34.9164, 10) (-120, -36, 10) (-105.4726, -34.9164, 10) (-100.462, -30.5633, 10) (-90.0493, -20.9917, 10) (-99.0825, -8.7446, 10) (-100, 0, 0) (-99.0825, 8.7446, 0) (-90.0493, 20.9917, 0) (-100.462, 30.5633, 0) (-105.4726, 34.9164, 0) (-120, 36, 0) (-134.5274, 34.9164, 0) (-139.538, 30.5633, 0) (-149.9507, 20.9917, 0) (-140.9175, 8.7446, 0) (-140, 0, 0) (-140.9175, -8.7446, 0) (-149.9507, -20.9917, 0) (-139.538, -30.5633, 0) (-134.5274, -34.9164, 0) (-120, -36, 0) (-105.4726, -34.9164, 0) (-100.462, -30.5633, 0) (-90.0493, -20.9917, 0) (-99.0825, -8.7446, 0) on bodies 27 in component "rectangle4"
chamfer "Chamfer1'''''''''''''''" distance 1 angle 45 8 edges at (-105.594, -17.8303, 10) (-145.594, 22.1697, 10) (-145.594, -17.8303, 10) (-145.594, -22.1697, 0) (-105.594, -22.1697, 0) (-105.594, 17.8303, 0) (-105.594, 22.1697, 10) (-145.594, 17.8303, 0) on bodies 27 in component "rectangle4"
component "base" placed x (1, 0, 0) y (0, 1, 0) z (0, 0, 1) at (0, 0, 0)
component "pins" placed x (1, 0, 0) y (0, 1, 0) z (0, 0, 1) at (0, 0, 0)
component "square1" placed x (1, 0, 0) y (0, 1, 0) z (0, 0, 1) at (0, 0, 0)
component "square2" placed x (1, 0, 0) y (0, 1, 0) z (0, 0, 1) at (0, 0, 0)
component "square3" placed x (1, 0, 0) y (0, 1, 0) z (0, 0, 1) at (0, 0, 0)
component "square4" placed x (1, 0, 0) y (0, 1, 0) z (0, 0, 1) at (0, 0, 0)
component "circle1" placed x (1, 0, 0) y (0, 1, 0) z (0, 0, 1) at (0, 0, 0)
component "circle2" placed x (1, 0, 0) y (0, 1, 0) z (0, 0, 1) at (0, 0, 0)
component "circle3" placed x (1, 0, 0) y (0, 1, 0) z (0, 0, 1) at (0, 0, 0)
component "circle4" placed x (1, 0, 0) y (0, 1, 0) z (0, 0, 1) at (0, 0, 0)
component "triangle1" placed x (1, 0, 0) y (0, 1, 0) z (0, 0, 1) at (0, 0, 0)
component "triangle2" placed x (1, 0, 0) y (0, 1, 0) z (0, 0, 1) at (0, 0, 0)
component "triangle3" placed x (1, 0, 0) y (0, 1, 0) z (0, 0, 1) at (0, 0, 0)
component "triangle4" placed x (1, 0, 0) y (0, 1, 0) z (0, 0, 1) at (0, 0, 0)
component "rectangle1" placed x (1, 0, 0) y (0, 1, 0) z (0, 0, 1) at (0, 0, 0)
component "rectangle2" placed x (1, 0, 0) y (0, 1, 0) z (0, 0, 1) at (0, 0, 0)
component "rectangle3" placed x (1, 0, 0) y (0, 1, 0) z (0, 0, 1) at (0, 0, 0)
component "rectangle4" placed x (1, 0, 0) y (0, 1, 0) z (0, 0, 1) at (0, 0, 0)
equation "d1 = tileSize * 4"
equation "d2 = tileSize"
equation "d3 = tileSize * 2"
equation "d4 = tileSize"
equation "tileSize = 80 mm"
equation "pinThickness = 12 mm"
equation "d7 = pinThickness"
equation "d8 = tileSize / 2"
equation "d9 = pinThickness"
equation "pinDistance = 40 mm"
equation "d11 = pinDistance / 2"
equation "d26 = pinThickness"
equation "d27 = sqrt(2) * pinDistance / 2"
equation "baseRounding = 10 mm"
equation "baseChamfer = 1 mm"
equation "tileRounding = 10 mm"
equation "tileChamfer = 1 mm"
equation "d35 = baseRounding"
equation "d39 = baseChamfer"
equation "d43 = tileThickness"
equation "d50 = tileChamfer"
equation "d53 = tileChamfer"
equation "d54 = tileSize - tileSpacing * 2"
equation "tileSpacing = 4 mm"
equation "d56 = tileThickness"
equation "tileThickness = 10 mm"
equation "d59 = tileThickness"
equation "d61 = tileChamfer"
equation "d66 = tileSize + tileSpacing * 4"
equation "d67 = tileThickness"
equation "d70 = tileRounding"
equation "d71 = tileChamfer"
equation "d72 = tileThickness"
equation "d79 = tileSize / 2"
equation "d80 = tileSize - tileSpacing * 2"
equation "d81 = tileThickness"
equation "d83 = tileThickness"
equation "d86 = tileRounding"
equation "d87 = tileChamfer"
equation "d88 = tileChamfer"
equation "d89 = pinThickness"
equation "d90 = tan(30 deg) * pinDistance"
equation "d93 = tileSize - tileSpacing * 2"
equation "d94 = tileThickness"
equation "d96 = tileThickness"
equation "d98 = tileChamfer"
equation "d99 = tileChamfer"
equation "d102 = tileSize"
equation "d103 = tileSize"
equation "d104 = tileThickness"
equation "d106 = tileSpacing"
equation "d107 = tileThickness"
equation "d109 = tileThickness"
equation "d112 = tileRounding"
equation "d113 = tileChamfer"
equation "d114 = tileChamfer"
equation "d115 = tileSize - tileSpacing * 2"
equation "d116 = tileThickness"
equation "d118 = tileThickness"
equation "d120 = tileChamfer"
equation "d121 = tileChamfer"
equation "d126 = tileSize / 2"
equation "d127 = tileSize - tileSpacing * 2"
equation "d128 = tileThickness"
equation "d130 = tileThickness"
equation "d133 = tileRounding"
equation "d134 = tileChamfer"
equation "d135 = tileChamfer"
equation "d136 = tileSize / 2"
equation "d137 = tileSize - tileSpacing * 2"
equation "d138 = tileThickness"
equation "d144 = tileSpacing"
equation "d145 = tileThickness"
equation "d148 = tileRounding"
equation "d152 = tileRounding / 2"
equation "d153 = tileSize - tileSpacing * 2"
equation "d154 = tileSize - tileSpacing * 2"
equation "d155 = tileThickness"
equation "d157 = tileThickness"
equation "d160 = tileRounding"
equation "d161 = tileChamfer"
equation "d162 = tileChamfer"
equation "d163 = tileSize + tileSpacing * 4"
equation "d166 = tileThickness"
equation "d169 = tileRounding"
equation "d170 = tileThickness"
equation "d172 = tileSpacing"
equation "d173 = tileThickness"
equation "d176 = tileRounding / 2"
equation "d177 = tileChamfer"
equation "d178 = tileChamfer"
equation "d179 = tileSize - tileSpacing * 2"
equation "d180 = tileThickness"
equation "d182 = tileThickness"
equation "d184 = tileChamfer"
equation "d185 = tileChamfer"
equation "d186 = tileSize + tileSpacing * 4"
equation "d189 = tileThickness"
equation "d191 = tileThickness"
equation "d193 = tileSpacing"
equation "d194 = tileThickness"
equation "d197 = tileRounding"
equation "d199 = tileRounding / 2"
equation "d200 = tileChamfer"
equation "d201 = tileChamfer"
equation "d202 = tileSize - tileSpacing * 2"
equation "d203 = tileSize - tileSpacing * 2"
equation "d204 = tileThickness"
equation "d206 = tileThickness"
equation "d209 = tileRounding"
equation "d210 = tileChamfer"
equation "d211 = tileChamfer"
equation "d212 = tileSize + tileSpacing * 4"
equation "d215 = tileThickness"
equation "d217 = tileThickness"
equation "d220 = tileRounding"
equation "d221 = tileChamfer"
equation "d222 = tileChamfer"
equation "d223 = tileSize / 2"
equation "d224 = tileSize - tileSpacing * 2"
equation "d225 = tileThickness"
equation "d227 = tileThickness"
equation "d229 = tileSpacing"
equation "d230 = tileThickness"
equation "d233 = tileRounding"
equation "d235 = tileRounding / 2"
equation "d236 = tileChamfer"
equation "d237 = tileChamfer"
equation "d238 = tileSpacing"
equation "d239 = tileThickness"
equation "d242 = tileRounding / 2"
